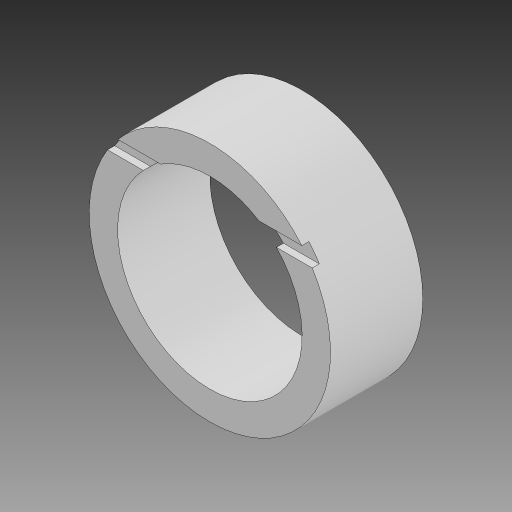
# Autodesk Inventor part: sonar
Saved by Autodesk Inventor 2023 (Build 270158000, 158)
## iProperties
Created: 2024-02-02
Part Number: sonar
Material: Všeobecné
Document SubType Name: Modeling
Designer: matej
Mass: 4.69986 g
Surface Area: 33.3362 cm^2
Volume: 4.69986 cm^3
Density: 1 g/cm^3
Appearance: Výchozí
Author: matej
Autodesk Inventor part; units mm, degrees
ref_plane "YZ Plane" through (0, 0, 0) normal (1, 0, 0) x (0, 1, 0)
ref_plane "XZ Plane" through (0, 0, 0) normal (0, 1, 0) x (-1, 0, 0)
ref_plane "XY Plane" through (0, 0, 0) normal (0, 0, 1) x (1, 0, 0)
sketch "Náčrt1" plane through (0, 0, 0) normal (0, 0, 1) x (1, 0, 0)
  circle A0 centre (0, 0) radius 17
  circle A1 centre (0, 0) radius 13
  dimension "d0" = 34
  dimension "d3" = 26
  constraints: 2 centre point, 2 coincident
  measures "d0" diameter of A0
  measures "d3" diameter of A1
extrude "Vysunutí1" add sketch "Náčrt1" along normal blind 13
sketch "Náčrt2" plane through (0, 0, 0) normal (1, 0, 0) x (0, 1, 0)
  line L0 (17, 0) -> (-17, 0) projected
  circle A0 centre (15, 0) radius 1.1
  line L1 (17, 13) -> (-17, 13) projected
  line L2 (17, 0) -> (-17, 0) projected
  line L3 (-13, 13) -> (13, 13) projected
  line L4 (-13, 0) -> (13, 0) projected
  line L5 (17, 0) -> (17, 13) projected
  line L6 (13, 13) -> (13, 0) projected
  line L7 (0, -4.32) -> (0, 18.22) projected
  point P0 (0, 0)
  point P1 (13.9, 0)
  point P2 (16.1, 0)
  dimension "d4" = 2.2
  dimension "d6" = 2
  dimension "d7" = 2
  constraints: 1 centre point, 1 point on line
  measures "d4" diameter of A0
  measures "d6" distance from line of L5 A0.centre
  measures "d7" distance from line of A0.centre L6
revolve "Rotace1" cut sketch "Náčrt2" angle 360 about axis through (0, 0, -10) along (0, 0, 1) picked at (15.2396, 0.5599) contours L0 A0
sketch "Náčrt4" plane through (0, 0, 13) normal (0, 0, 1) x (1, 0, 0)
  line L0 (-17, 11) -> (17, 11)
  line L1 (17, 11) -> (17, 9)
  line L2 (17, 9) -> (-17, 9)
  line L3 (-17, 9) -> (-17, 11)
  line L4 (-17, 11) -> (17, 9) construction
  line L5 (17, 11) -> (-17, 9) construction
  point P0 (0, 0)
  point P1 (0, 10)
  dimension "d9" = 2
  dimension "d10" = 34
  dimension "d11" = 10
  constraints: 12 end point, 2 midpoint, 2 parallel, 1 horizontal, 1 perpendicular, 1 vertical alignment
  measures "d9" distance of L0.end L1.end
  measures "d10" distance of L0.start L0.end
  measures "d11" distance of point (0, 0) point (0, 10)
extrude "Vysunutí2" cut sketch "Náčrt4" against normal blind 1
